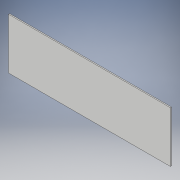
# Autodesk Inventor part: Drive Side Plates
Saved by Autodesk Inventor 2017 (Build 210142000, 142)
## iProperties
Created: 2017-10-12
Part Number: Drive Side Plates
Material: Generic
Document SubType Name: Modeling
Designer: Kenneth
Density: 1 g/cm^3
Appearance: Default
Author: Kenneth
Autodesk Inventor part; units mm, degrees
ref_plane "YZ Plane" through (0, 0, 0) normal (1, 0, 0) x (0, 1, 0)
ref_plane "XZ Plane" through (0, 0, 0) normal (0, 1, 0) x (-1, 0, 0)
ref_plane "XY Plane" through (0, 0, 0) normal (0, 0, 1) x (1, 0, 0)
sketch "Sketch1" plane through (0, 0, 0) normal (0, 0, 1) x (1, 0, 0)
  line L0 (-222.25, -69.85) -> (222.25, -69.85)
  line L1 (222.25, -69.85) -> (222.25, 69.85)
  line L2 (222.25, 69.85) -> (-222.25, 69.85)
  line L3 (-222.25, 69.85) -> (-222.25, -69.85)
  line L4 (-222.25, -69.85) -> (222.25, 69.85) construction
  line L5 (222.25, -69.85) -> (-222.25, 69.85) construction
  point P0 (0, 0)
  dimension "d0" = 444.5
  dimension "d1" = 139.7
  constraints: 12 end point, 2 midpoint, 2 parallel, 1 horizontal, 1 perpendicular
  measures "d0" distance of L1.end L2.end
  measures "d1" distance of L0.end L1.end
extrude "Extrusion1" add sketch "Sketch1" along normal blind 3.175
body "Solid1"
